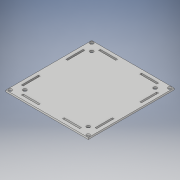
# Autodesk Inventor part: Part Buttom
Saved by Autodesk Inventor 2019 (Build 230136000, 136)
## iProperties
Created: 2019-07-08
Part Number: Part Buttom
Material: Generic
Document SubType Name: Modeling
Designer: azriel
Density: 1 g/cm^3
Appearance: Default
Author: azriel
Autodesk Inventor part; units mm, degrees
ref_plane "YZ Plane" through (0, 0, 0) normal (1, 0, 0) x (0, 1, 0)
ref_plane "XZ Plane" through (0, 0, 0) normal (0, 1, 0) x (-1, 0, 0)
ref_plane "XY Plane" through (0, 0, 0) normal (0, 0, 1) x (1, 0, 0)
sketch "Sketch1" plane through (0, 0, 0) normal (0, 1, 0) x (-1, 0, 0)
  line L0 (86.8555, -89.5803) -> (86.8555, 160.4197)
  line L1 (86.8555, 160.4197) -> (-153.1445, 160.4197)
  line L2 (-153.1445, 160.4197) -> (-153.1445, -89.5803)
  line L3 (-153.1445, -89.5803) -> (86.8555, -89.5803)
  line L4 (-143.1445, 125.4197) -> (-143.1445, 75.4197)
  line L5 (-143.1445, 75.4197) -> (-138.1445, 75.4197)
  line L6 (-138.1445, 75.4197) -> (-138.1445, 125.4197)
  line L7 (-138.1445, 125.4197) -> (-143.1445, 125.4197)
  line L8 (-138.1445, -54.5803) -> (-138.1445, -4.5803)
  line L9 (-138.1445, -4.5803) -> (-143.1445, -4.5803)
  line L10 (-143.1445, -4.5803) -> (-143.1445, -54.5803)
  line L11 (-143.1445, -54.5803) -> (-138.1445, -54.5803)
  line L12 (-118.1445, -74.5803) -> (-68.1445, -74.5803)
  line L13 (-68.1445, -74.5803) -> (-68.1445, -79.5803)
  line L14 (-68.1445, -79.5803) -> (-118.1445, -79.5803)
  line L15 (-118.1445, -79.5803) -> (-118.1445, -74.5803)
  line L16 (1.8555, -74.5803) -> (51.8555, -74.5803)
  line L17 (51.8555, -74.5803) -> (51.8555, -79.5803)
  line L18 (51.8555, -79.5803) -> (1.8555, -79.5803)
  line L19 (1.8555, -79.5803) -> (1.8555, -74.5803)
  line L20 (71.8555, -54.5803) -> (71.8555, -4.5803)
  line L21 (71.8555, -4.5803) -> (76.8555, -4.5803)
  line L22 (76.8555, -4.5803) -> (76.8555, -54.5803)
  line L23 (76.8555, -54.5803) -> (71.8555, -54.5803)
  line L24 (76.8555, 75.4197) -> (76.8555, 125.4197)
  line L25 (76.8555, 125.4197) -> (71.8555, 125.4197)
  line L26 (71.8555, 125.4197) -> (71.8555, 75.4197)
  line L27 (71.8555, 75.4197) -> (76.8555, 75.4197)
  line L28 (51.8555, 145.4197) -> (1.8555, 145.4197)
  line L29 (1.8555, 145.4197) -> (1.8555, 150.4197)
  line L30 (1.8555, 150.4197) -> (51.8555, 150.4197)
  line L31 (51.8555, 150.4197) -> (51.8555, 145.4197)
  line L32 (-68.1445, 145.4197) -> (-118.1445, 145.4197)
  line L33 (-118.1445, 145.4197) -> (-118.1445, 150.4197)
  line L34 (-118.1445, 150.4197) -> (-68.1445, 150.4197)
  line L35 (-68.1445, 150.4197) -> (-68.1445, 145.4197)
  circle A0 centre (59.3555, -62.0803) radius 5
  circle A1 centre (-125.6445, -62.0803) radius 5
  circle A2 centre (59.3555, 132.9197) radius 5
  circle A3 centre (-125.6445, 132.9197) radius 5
  line L36 (76.8555, -89.5803) -> (86.8555, -89.5803)
  line L37 (86.8555, -89.5803) -> (86.8555, -79.5803)
  line L38 (86.8555, -77.0803) -> (86.8555, -89.5803)
  line L39 (86.8555, -89.5803) -> (74.3555, -89.5803)
  circle A4 centre (80.6055, -83.3303) radius 5
  line L40 (-153.1445, -77.0803) -> (-153.1445, -89.5803)
  line L41 (-153.1445, -89.5803) -> (-140.6445, -89.5803)
  circle A5 centre (-146.8945, -83.3303) radius 5
  line L42 (-140.6445, 160.4197) -> (-153.1445, 160.4197)
  line L43 (-153.1445, 160.4197) -> (-153.1445, 147.9197)
  circle A6 centre (-146.8945, 154.1697) radius 5
  line L44 (74.3555, 160.4197) -> (86.8555, 160.4197)
  line L45 (86.8555, 160.4197) -> (86.8555, 147.9197)
  circle A7 centre (80.6055, 154.1697) radius 5
  point P0 (0, 0)
  dimension "d0" = 250
  dimension "d1" = 240
  dimension "d4" = 35
  dimension "d5" = 10
  dimension "d8" = 10
  dimension "d9" = 35
  dimension "d12" = 10
  dimension "d13" = 35
  dimension "d19" = 10
  dimension "d20" = 10
  dimension "d23" = 10
  dimension "d25" = 5
  dimension "d26" = 10
  dimension "d30" = 35
  dimension "d31" = 35
  dimension "d32" = 35
  dimension "d37" = 10
  dimension "d40" = 10
  dimension "d43" = 10
  dimension "d46" = 10
  dimension "d49" = 10
  dimension "d50" = 10
  dimension "d51" = 10
  dimension "d52" = 10
  constraints: 92 end point, 18 parallel, 9 perpendicular, 8 centre point, 5 point on line, 5 vertical, 4 horizontal
  measures "d0" distance of L0.start L0.end
  measures "d1" distance of L1.end L0.end
  measures "d4" distance between parallel lines of L1 L7
  measures "d5" distance between parallel lines of L2 L4
  measures "d8" distance between parallel lines of L2 L10
  measures "d9" distance between parallel lines of L11 L3
  measures "d12" distance between parallel lines of L14 L3
  measures "d13" distance between parallel lines of L2 L15
  measures "d19" distance between parallel lines of L0 L22
  measures "d20" distance between parallel lines of L0 L24
  measures "d23" distance between parallel lines of L1 L30
  measures "d25" distance between parallel lines of L12 L14
  measures "d26" distance between parallel lines of L18 L3
  measures "d30" distance from line of L2 L32.end
  measures "d31" distance from line of L20.start L3
  measures "d32" distance between parallel lines of L1 L25
  measures "d37" diameter of A0
  measures "d40" diameter of A1
  measures "d43" diameter of A2
  measures "d46" diameter of A3
  measures "d49" diameter of A4
  measures "d50" diameter of A5
  measures "d51" diameter of A6
  measures "d52" diameter of A7
extrude "Extrusion3" add sketch "Sketch1" along normal blind 5
body "Solid3"
